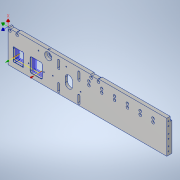
# Autodesk Inventor part: Frame Back
Saved by Autodesk Inventor 2020 (Build 240168000, 168)
## iProperties
Created: 2019-01-21
Part Number: Frame Back
Material: Aluminum 6061
Document SubType Name: Modeling
Designer: LillaHunden
Density: 2.7 g/cm^3
Appearance: Aluminum - Flat
Author: LillaHunden
Autodesk Inventor part; units mm, degrees
ref_plane "YZ Plane" through (0, 0, 0) normal (1, 0, 0) x (0, 1, 0)
ref_plane "XZ Plane" through (0, 0, 0) normal (0, 1, 0) x (-1, 0, 0)
sketch "Sketch1" plane through (0, 0, 0) normal (0, 0, 1) x (1, 0, 0)
  line L0 (-165.2266, -26.9823) -> (205.7734, -26.9823)
  line L1 (205.7734, -26.9823) -> (205.7734, -103.9647)
  line L2 (205.7734, -103.9647) -> (-165.2266, -103.9647)
  line L3 (-165.2266, -103.9647) -> (-165.2266, -26.9823)
  line L4 (15.7734, -103.9647) -> (41.2734, -103.9647) construction
  point P0 (0, 0)
  point P1 (20.2734, -103.9647)
  constraints: 8 end point, 2 parallel, 1 horizontal, 1 horizontal alignment, 1 midpoint, 1 perpendicular
extrude "Extrusion1" add sketch "Sketch1" along normal blind 12
sketch "Sketch2" plane through (-165.2266, -103.9647, 0) normal (-1, 0, 0) x (0, 0, 1)
  line L0 (0, 0) -> (0, 76.9823) construction
  line L1 (0, 0) -> (12, 0) projected
  line L2 (12, 76.9823) -> (12, 0) construction
  line L3 (0, 76.9823) -> (12, 76.9823) construction
  line L4 (4, 67) -> (-280, 67) construction
  line L5 (4, 67) -> (4, 76.9823) construction
  line L6 (-280, 76.9823) -> (4, 76.9823) construction
  line L7 (0, 103.9647) -> (4, 103.9647)
  line L8 (4, 103.9647) -> (4, 67)
  line L9 (4, 67) -> (0, 67)
  line L10 (0, 67) -> (0, 103.9647)
  line L11 (-280, 76.9823) -> (-280, 67) projected
  constraints: 8 end point, 2 parallel, 1 horizontal, 1 perpendicular, 1 other
extrude "Extrusion2" cut sketch "Sketch2" against normal through all
sketch "Sketch3" plane through (0, 0, 0) normal (0, 0, -1) x (-1, 0, 0)
  circle A0 centre (71.5266, -39.9823) radius 2.5 construction
  arc A1 (66.419, -43.1308) -> (56.0091, -36.9647) centre (56.0091, -48.8349) ccw
  line L0 (165.2266, -36.9647) -> (-205.7734, -36.9647) construction
  line L1 (71.5266, -34.9823) -> (71.5266, -45.9823) construction
  arc A2 (87.044, -36.9647) -> (76.6341, -43.1308) centre (87.044, -48.8349) ccw
  line L2 (56.0091, -36.9647) -> (87.044, -36.9647)
  arc A3 (66.419, -43.1308) -> (76.6341, -43.1308) centre (71.5266, -39.9823) ccw
  arc A4 (75.5133, -36.9647) -> (67.5399, -36.9647) centre (71.5266, -39.9823) ccw construction
  point P0 (0, 0)
  dimension "d9" = 6
  constraints: 10 point on circle, 5 centre point, 4 end point, 3 point on line, 3 symmetric about line, 2 tangent, 1 coincident, 1 collinear, 1 other
  measures "d9" radius of A3
extrude "Extrusion3" cut sketch "Sketch3" against normal up to surface (4 mm away)
sketch "Sketch4" plane through (0, 0, 0) normal (0, 0, -1) x (-1, 0, 0)
  circle A0 centre (23.2266, -67.9647) radius 18.9 projected
  circle A1 centre (23.2266, -67.9647) radius 19.5 projected
  point P0 (0, 0)
extrude "Extrusion4" cut sketch "Sketch4" against normal blind 6.25 contours A0 | A1
sketch "Sketch5" plane through (-23.2266, -67.9647, 6.25) normal (0, 0, -1) x (-1, 0, 0)
  circle A0 centre (0, 0) radius 2.5 projected
  circle A1 centre (0, 0) radius 3.5
  point P0 (-23.2266, 67.9647)
  dimension "d15" = 1
  constraints: 1 centre point
  measures "d15" radial gap between concentric circles of A0 A1
extrude "Extrusion5" cut sketch "Sketch5" against normal through all contours A0 | A1
sketch "Sketch6" plane through (0, 0, 0) normal (0, 0, -1) x (-1, 0, 0)
  circle A0 centre (-0.3434, -44.3947) radius 2.6 projected
  circle A1 centre (46.7966, -44.3947) radius 2.6 projected
  circle A2 centre (46.7966, -91.5347) radius 2.6 projected
  circle A3 centre (-0.3434, -91.5347) radius 2.6 projected
  point P0 (0, 0)
hole "Hole1" at (0.3434, -91.5347, 0) at (-46.7966, -91.5347, 0) at (0.3434, -44.3947, 0) at (-46.7966, -44.3947, 0) direction (0, 0, 1) diameter 4.134 depth 14.2 thread size "M5x0.8" class "6H" standard "ISO Metric profile"
chamfer "Chamfer3" distance 0.2 angle 45 8 edges at (0.3434, -46.4617, 12) (-46.7966, -46.4617, 12) (-46.7966, -93.6017, 12) (0.3434, -93.6017, 12) (0.3434, -93.6017, 0) (-46.7966, -93.6017, 0) (-46.7966, -46.4617, 0) (0.3434, -46.4617, 0)
sketch "Sketch7" plane through (-165.2266, -36.9647, 4) normal (0, 0, -1) x (-1, 0, 0)
  circle A0 centre (-93.7, -3.0177) radius 4.7625 projected
  circle A1 centre (-93.7, -3.0177) radius 4.7125
  point P0 (-165.2266, 36.9647)
  dimension "d31" = 0.05
  constraints: 1 centre point
  measures "d31" radial gap between concentric circles of A0 A1
extrude "Extrusion6" cut sketch "Sketch7" against normal through all contours A0 | A1
chamfer "Chamfer4" distance 0.5 angle 45 2 edges at (-66.7641, -39.9823, 4) (-66.7641, -39.9823, 12)
sketch "Sketch8" plane through (-165.2266, -36.9647, 4) normal (0, 0, -1) x (-1, 0, 0)
  line L0 (-18, 6.4823) -> (-7, 6.4823) construction
  line L1 (-7, 6.4823) -> (-7, 10.6239) construction
  line L2 (-18, 10.6239) -> (-18, 6.4823) construction
  line L3 (-19, 7.9823) -> (-6, 7.9823) projected
  line L4 (-19, 9.9823) -> (-19, 7.9823) projected
  line L5 (-6, 7.9823) -> (-6, 9.9823) projected
  arc A0 (-21.8284, 9.9823) -> (-19, 7.9823) centre (-19, 10.9823) ccw
  line L6 (-371, 9.9823) -> (0, 9.9823) projected
  line L7 (-21.8284, 9.9823) -> (-6, 9.9823)
  line L8 (-12.5, 7.9823) -> (-12.5, 13.9823)
  arc A1 (-6, 7.9823) -> (-3.1716, 9.9823) centre (-6, 10.9823) ccw
  line L9 (-3.1716, 9.9823) -> (-6, 9.9823)
  point P0 (-165.2266, 36.9647)
  dimension "d37" = 6
  constraints: 6 end point, 5 point on circle, 4 point on line, 2 centre point, 1 collinear, 1 midpoint, 1 perpendicular, 1 symmetric about line, 1 tangent, 1 vertical, 1 other
  measures "d37" diameter of A0
extrude "Extrusion7" cut sketch "Sketch8" against normal through all
sketch "Sketch9" plane through (-165.2266, -36.9647, 4) normal (0, 0, -1) x (-1, 0, 0)
  line L0 (-209, 9.9823) -> (-209, 7.9823) projected
  line L1 (-209, 7.9823) -> (-196, 7.9823) projected
  line L2 (-196, 7.9823) -> (-196, 9.9823) projected
  line L3 (-190, 9.9823) -> (-196, 9.9823) projected
  line L4 (-190, 0) -> (-190, 9.9823) projected
  line L5 (-215, 0) -> (-190, 0) projected
  line L6 (-215, 0) -> (-215, 9.9823) projected
  line L7 (-209, 9.9823) -> (-215, 9.9823) projected
  arc A0 (-211.8284, 9.9823) -> (-209, 7.9823) centre (-209, 10.9823) ccw
  line L8 (-202.5, 7.9823) -> (-202.5, 9.9823) construction
  arc A1 (-196, 7.9823) -> (-193.1716, 9.9823) centre (-196, 10.9823) ccw
  line L9 (-371, 9.9823) -> (-21.8284, 9.9823) projected
  line L10 (-211.8284, 9.9823) -> (-193.1716, 9.9823)
  point P0 (-165.2266, 36.9647)
  dimension "d40" = 6
  constraints: 5 end point, 5 point on circle, 3 point on line, 2 centre point, 2 midpoint, 1 symmetric about line, 1 tangent, 1 vertical, 1 other
  measures "d40" diameter of A0
extrude "Extrusion8" cut sketch "Sketch9" against normal through all contours L9 L2 L1 L0 | L0 A0 L7 | L3 A1 L2
sketch "Sketch10" plane through (0, 0, 0) normal (0, 0, -1) x (-1, 0, 0)
  circle A0 centre (23.2266, -67.9647) radius 3.5 construction
  line L0 (23.2266, -75.9647) -> (23.2266, -59.9647) construction
  line L1 (3.7266, -75.9647) -> (3.7266, -59.9647)
  line L2 (42.7266, -59.9647) -> (42.7266, -75.9647)
  arc A1 (3.7266, -75.9647) -> (42.7266, -75.9647) centre (23.2266, -75.9647) ccw
  arc A2 (42.7266, -59.9647) -> (3.7266, -59.9647) centre (23.2266, -59.9647) ccw
  circle A3 centre (23.2266, -67.9647) radius 3.5 construction
  circle A4 centre (23.2266, -67.9647) radius 19.5 construction
  line L3 (56.0091, -36.9647) -> (-205.7734, -36.9647) construction
  point P0 (0, 0)
  dimension "d43" = 8
  constraints: 8 end point, 5 tangent, 4 point on circle, 2 centre point, 1 midpoint, 1 parallel, 1 vertical
  measures "d43" distance of L0.end A0.centre
extrude "Extrusion9" cut sketch "Sketch10" against normal up to surface (6.25 mm away)
sketch "Sketch11" plane through (0, 0, 0) normal (0, 0, -1) x (-1, 0, 0)
  line L0 (-0.3434, -36.3947) -> (-0.3434, -52.3947) construction
  line L1 (-2.9434, -36.3947) -> (-2.9434, -52.3947)
  line L2 (2.2566, -52.3947) -> (2.2566, -36.3947)
  arc A0 (2.2566, -36.3947) -> (-2.9434, -36.3947) centre (-0.3434, -36.3947) ccw
  arc A1 (-2.9434, -52.3947) -> (2.2566, -52.3947) centre (-0.3434, -52.3947) ccw
  circle A2 centre (-0.3434, -44.3947) radius 2.067 construction
  circle A3 centre (46.7966, -44.3947) radius 2.267 construction
  line L3 (56.0091, -36.9647) -> (-205.7734, -36.9647) construction
  line L4 (46.7966, -36.3947) -> (46.7966, -52.3947) construction
  line L5 (44.1966, -36.3947) -> (44.1966, -52.3947)
  line L6 (49.3966, -52.3947) -> (49.3966, -36.3947)
  arc A4 (49.3966, -36.3947) -> (44.1966, -36.3947) centre (46.7966, -36.3947) ccw
  arc A5 (44.1966, -52.3947) -> (49.3966, -52.3947) centre (46.7966, -52.3947) ccw
  line L7 (-0.3434, -83.5347) -> (-0.3434, -99.5347) construction
  line L8 (-2.9434, -83.5347) -> (-2.9434, -99.5347)
  line L9 (2.2566, -99.5347) -> (2.2566, -83.5347)
  arc A6 (2.2566, -83.5347) -> (-2.9434, -83.5347) centre (-0.3434, -83.5347) ccw
  arc A7 (-2.9434, -99.5347) -> (2.2566, -99.5347) centre (-0.3434, -99.5347) ccw
  line L10 (46.7966, -83.5347) -> (46.7966, -99.5347) construction
  line L11 (44.1966, -83.5347) -> (44.1966, -99.5347)
  line L12 (49.3966, -99.5347) -> (49.3966, -83.5347)
  arc A8 (49.3966, -83.5347) -> (44.1966, -83.5347) centre (46.7966, -83.5347) ccw
  arc A9 (44.1966, -99.5347) -> (49.3966, -99.5347) centre (46.7966, -99.5347) ccw
  point P0 (0, 0)
  point P1 (46.7966, -44.3947)
  point P2 (46.7966, -44.3947)
  point P3 (-0.3434, -91.5347)
  point P4 (-0.3434, -91.5347)
  point P5 (46.7966, -91.5347)
  point P6 (46.7966, -91.5347)
  dimension "d46" = 8
  dimension "d47" = 5.2
  dimension "d50" = 47.14
  dimension "d53" = 47.14
  constraints: 32 end point, 16 point on circle, 8 centre point, 4 coincident, 4 tangent, 2 vertical, 1 collinear, 1 horizontal, 1 midpoint, 1 parallel, 38 other
  measures "d46" distance of point (-0.343, -44.395) L0.end
  measures "d47" diameter of A1
  measures "d50" distance of L1.start L5.start
  measures "d53" distance of L1.start L8.start
extrude "Extrusion10" cut sketch "Sketch11" against normal through all
sketch "Sketch12" plane through (0, 0, 6.25) normal (0, 0, -1) x (-1, 0, 0)
  circle A0 centre (23.2266, -67.9647) radius 3.5 construction
  line L0 (23.2266, -75.9647) -> (23.2266, -59.9647) construction
  circle A1 centre (23.2266, -67.9647) radius 3.5 construction
  line L1 (19.7266, -75.9647) -> (19.7266, -59.9647)
  line L2 (26.7266, -59.9647) -> (26.7266, -75.9647)
  arc A2 (19.7266, -75.9647) -> (26.7266, -75.9647) centre (23.2266, -75.9647) ccw
  arc A3 (26.7266, -59.9647) -> (19.7266, -59.9647) centre (23.2266, -59.9647) ccw
  point P0 (0, 0)
  dimension "d58" = 8
  constraints: 8 end point, 4 point on circle, 4 tangent, 2 centre point, 1 midpoint, 1 parallel, 1 vertical
  measures "d58" distance of A1.centre L0.end
extrude "Extrusion11" cut sketch "Sketch12" against normal through all
sketch "Sketch13" plane through (0, 0, 12) normal (0, 0, 1) x (1, 0, 0)
  line L0 (-146.2266, -26.9823) -> (-146.2266, -28.9823) construction
  line L1 (-146.2266, -28.9823) -> (-159.2266, -28.9823) construction
  line L2 (-159.2266, -28.9823) -> (-159.2266, -26.9823) construction
  line L3 (-165.2266, -26.9823) -> (-159.2266, -26.9823) construction
  line L4 (-165.2266, -36.9647) -> (-165.2266, -26.9823) construction
  line L5 (-140.2266, -36.9647) -> (-165.2266, -36.9647) construction
  line L6 (-140.2266, -36.9647) -> (-140.2266, -26.9823) construction
  line L7 (-146.2266, -26.9823) -> (-140.2266, -26.9823) construction
  line L8 (43.7734, -26.9823) -> (43.7734, -28.9823) construction
  line L9 (43.7734, -28.9823) -> (30.7734, -28.9823) construction
  line L10 (30.7734, -28.9823) -> (30.7734, -26.9823) construction
  line L11 (24.7734, -26.9823) -> (30.7734, -26.9823) construction
  line L12 (24.7734, -36.9647) -> (24.7734, -26.9823) construction
  line L13 (49.7734, -36.9647) -> (24.7734, -36.9647) construction
  line L14 (49.7734, -36.9647) -> (49.7734, -26.9823) construction
  line L15 (43.7734, -26.9823) -> (49.7734, -26.9823) construction
  circle A0 centre (-161.2266, -33.2125) radius 1.621 projected
  circle A1 centre (-144.2266, -33.2125) radius 1.621 projected
  point P0 (0, 0)
  point P1 (-161.2266, -33.2125)
  point P2 (-144.2266, -33.2125)
  point P3 (28.7734, -33.2125)
  point P4 (45.7734, -33.2125)
  dimension "d61" = 4
  dimension "d62" = 4
  dimension "d63" = 4
  dimension "d64" = 4
  constraints: 3 horizontal alignment
  measures "d61" distance from line of L4 point (-161.227, -33.213)
  measures "d62" distance from line of L6 point (-144.227, -33.213)
  measures "d63" distance from line of L12 point (28.773, -33.213)
  measures "d64" distance from line of L14 point (45.773, -33.213)
hole "Hole2" at (-161.2266, -33.2125, 12) at (-144.2266, -33.2125, 12) at (28.7734, -33.2125, 12) at (45.7734, -33.2125, 12) direction (0, 0, -1) diameter 3.4 depth 14.2 counterbore diameter 6.5 counterbore depth 3.4 clearance for "Socket Head Cap Screw ISO 4762" size "M3" standard "ISO"
sketch "Sketch14" plane through (0, 0, 12) normal (0, 0, 1) x (1, 0, 0)
  circle A0 centre (77.1068, -51.298) radius 1.621 construction
  circle A1 centre (173.6068, -51.298) radius 1.621 construction
  line L0 (108.2734, -36.9647) -> (108.2734, -41.9647) construction
  line L1 (108.2734, -41.9647) -> (93.2734, -41.9647) construction
  line L2 (93.2734, -41.9647) -> (93.2734, -36.9647) construction
  line L3 (12.7734, -36.9647) -> (93.2734, -36.9647) construction
  line L4 (12.7734, -55.9647) -> (12.7734, -36.9647) construction
  line L5 (205.7734, -55.9647) -> (12.7734, -55.9647) construction
  line L6 (205.7734, -55.9647) -> (205.7734, -36.9647) construction
  line L7 (108.2734, -36.9647) -> (205.7734, -36.9647) construction
  circle A2 centre (23.6068, -43.298) radius 1.621 projected
  circle A3 centre (53.6068, -51.298) radius 1.621 projected
  circle A4 centre (83.6068, -51.298) radius 1.621 projected
  circle A5 centre (113.6068, -43.298) radius 1.621 projected
  circle A6 centre (143.6068, -51.298) radius 1.621 projected
  circle A7 centre (173.6068, -43.298) radius 1.621 projected
  circle A8 centre (143.6068, -43.298) radius 1.621 projected
  circle A9 centre (113.6068, -51.298) radius 1.621 projected
  circle A10 centre (83.6068, -43.298) radius 1.621 projected
  circle A11 centre (53.6068, -43.298) radius 1.621 projected
  circle A12 centre (23.6068, -51.298) radius 1.621 projected
  point P0 (0, 0)
  point P1 (173.6068, -43.298)
  point P2 (143.6068, -51.298)
  point P3 (113.6068, -51.298)
  point P4 (83.6068, -51.298)
  point P5 (53.6068, -51.298)
  point P6 (23.6068, -51.298)
  point P7 (173.6068, -43.298)
  point P8 (143.6068, -43.298)
  point P9 (113.6068, -43.298)
  point P10 (83.6068, -43.298)
  point P11 (53.6068, -43.298)
  point P12 (23.6068, -43.298)
  dimension "d81" = 30
  dimension "d84" = 8
  constraints: 1 horizontal, 1 vertical, 11 other
  measures "d81" distance of A1.centre point (143.607, -51.298)
  measures "d84" distance of A1.centre point (173.607, -43.298)
hole "Hole3" at (173.6068, -43.298, 12) at (173.6068, -51.298, 12) at (143.6068, -51.298, 12) at (143.6068, -43.298, 12) at (113.6068, -51.298, 12) at (113.6068, -43.298, 12) at (83.6068, -43.298, 12) at (83.6068, -51.298, 12) at (53.6068, -51.298, 12) at (53.6068, -43.298, 12) at (23.6068, -51.298, 12) at (23.6068, -43.298, 12) direction (0, 0, -1) diameter 3.242 end through all counterbore diameter 6.5 counterbore depth 3.4 thread size "M4x0.7" class "6H" standard "ISO Metric profile"
sketch "Sketch15" plane through (0, 0, 0) normal (0, 0, -1) x (-1, 0, 0)
  line L0 (51.2266, -42.9647) -> (51.2266, -92.9647) construction
  line L1 (-4.7734, -92.9647) -> (-4.7734, -42.9647) construction
  line L2 (-1.7734, -39.9647) -> (48.2266, -39.9647) construction
  line L3 (-1.7734, -38.9647) -> (48.2266, -38.9647) construction
  line L4 (-5.7734, -92.9647) -> (-5.7734, -42.9647) construction
  line L5 (-10.1867, -31.4447) -> (56.6399, -31.4447)
  line L6 (56.6399, -31.4447) -> (56.6399, -107.0786)
  line L7 (56.6399, -107.0786) -> (-10.1867, -107.0786)
  line L8 (-10.1867, -107.0786) -> (-10.1867, -31.4447)
  line L9 (23.2266, -38.9647) -> (23.2266, -140.4412) construction
  line L10 (-205.7734, -103.9647) -> (165.2266, -103.9647) construction
  point P0 (0, 0)
  dimension "d87" = 1
  dimension "d88" = 1
  constraints: 14 end point, 4 parallel, 2 perpendicular, 1 horizontal, 1 midpoint, 1 other
  measures "d87" distance between parallel lines of L2 L3
  measures "d88" distance between parallel lines of L1 L4
extrude "Extrusion12" cut sketch "Sketch15" against normal blind 4
sketch "Sketch16" plane through (0, 0, 12) normal (0, 0, 1) x (1, 0, 0)
  arc A0 (-19.7266, -59.9647) -> (-26.7266, -59.9647) centre (-23.2266, -59.9647) ccw construction
  arc A1 (-26.7266, -75.9647) -> (-19.7266, -75.9647) centre (-23.2266, -75.9647) ccw construction
  circle A2 centre (-23.2266, -67.9647) radius 8 construction
  circle A3 centre (-23.2266, -67.9647) radius 8.6 construction
  line L0 (-23.2266, -53.9647) -> (-23.2266, -81.9647) construction
  line L1 (-31.8266, -62.5647) -> (-31.8266, -73.3647)
  line L2 (-14.6266, -73.3647) -> (-14.6266, -62.5647)
  arc A4 (-14.6266, -62.5647) -> (-31.8266, -62.5647) centre (-23.2266, -62.5647) ccw
  arc A5 (-31.8266, -73.3647) -> (-14.6266, -73.3647) centre (-23.2266, -73.3647) ccw
  arc A6 (-19.7266, -59.9647) -> (-26.7266, -59.9647) centre (-23.2266, -59.9647) ccw projected
  point P0 (0, 0)
  point P1 (-23.2266, -67.9647)
  point P2 (-23.2266, -79.4647)
  point P3 (-23.2266, -56.4647)
  dimension "d91" = 0.6
  dimension "d92" = 2.5
  dimension "d93" = 2.5
  constraints: 8 end point, 8 point on circle, 4 point on line, 4 tangent, 3 centre point, 1 midpoint, 1 parallel, 1 vertical
  measures "d91" radial gap between concentric circles of A2 A3
  measures "d92" distance of point (-23.227, -79.465) L0.end
  measures "d93" distance of point (-23.227, -56.465) L0.start
extrude "Extrusion13" cut sketch "Sketch16" against normal through all
sketch "Sketch17" plane through (0, 0, 12) normal (0, 0, 1) x (1, 0, 0)
  circle A0 centre (-71.5266, -39.9823) radius 8 construction
  circle A1 centre (-71.5266, -39.9823) radius 8.6
  point P0 (0, 0)
  dimension "d96" = 0.6
  constraints: 1 centre point
  measures "d96" radial gap between concentric circles of A0 A1
ref_plane "Work Plane1" through (-31.4029, -76.141, 6) normal (0, 0, -1) x (0.1439331, 0.9895874, 0)
extrude "Extrusion14" cut sketch "Sketch17" against normal up to surface (6 mm away)
sketch "Sketch18" plane through (-143.3981, -26.9823, 12) normal (0, 1, 0) x (1, 0, 0)
  line L0 (79.8716, -13.2) -> (63.8716, -13.2) construction
  line L1 (71.8716, -13.2) -> (71.8716, 7.5) construction
  line L2 (67.1091, 7.5) -> (76.6341, 7.5) construction
  line L3 (70.8561, 2.5) -> (71.8716, 2.5) construction
  circle A0 centre (71.8716, 2.5) radius 2
  line L4 (68.3716, 4) -> (68.3716, 1) projected
  point P0 (143.3981, 12)
  dimension "d99" = 4
  constraints: 4 end point, 2 midpoint, 1 centre point, 1 coincident, 1 perpendicular, 1 point on line
  measures "d99" diameter of A0
extrude "Extrusion15" cut sketch "Sketch18" against normal up to next
sketch "Sketch19" plane through (205.7734, -103.9647, 12) normal (1, 0, 0) x (0, 0, -1)
  point P0 (4.05, 68.9823)
  point P1 (4.05, 58.9823)
  point P2 (4.05, 43.4912)
  point P3 (4.05, 33.4912)
  point P4 (4.05, 18)
  point P5 (4.05, 8)
hole "Hole4" at (205.7734, -34.9823, 7.95) at (205.7734, -44.9823, 7.95) at (205.7734, -60.4735, 7.95) at (205.7734, -70.4735, 7.95) at (205.7734, -85.9647, 7.95) at (205.7734, -95.9647, 7.95) direction (-1, 0, 0) diameter 2.459 depth 8 tip angle 120 thread size "M3x0.5" class "6H" standard "ISO Metric profile"
sketch "Sketch20" plane through (-165.2266, -103.9647, 12) normal (-1, 0, 0) x (0, 0, 1)
  point P0 (-4.05, 58.9823)
  point P1 (-4.05, 43.4912)
  point P2 (-4.05, 33.4912)
  point P3 (-4.05, 18)
  point P4 (-4.05, 8)
hole "Hole6" at (-165.2266, -44.9823, 7.95) at (-165.2266, -60.4735, 7.95) at (-165.2266, -70.4735, 7.95) at (-165.2266, -85.9647, 7.95) at (-165.2266, -95.9647, 7.95) direction (1, 0, 0) diameter 2.459 depth 8 tip angle 120 thread size "M3x0.5" class "6H" standard "ISO Metric profile"
sketch "Sketch21" plane through (0, 0, 12) normal (0, 0, 1) x (1, 0, 0)
  line L0 (-110.2766, -61.1147) -> (-88.5766, -61.1147) construction
  line L1 (-85.5766, -64.1147) -> (-85.5766, -90.4147) construction
  arc A0 (-85.5766, -64.1147) -> (-88.5766, -61.1147) centre (-88.5766, -64.1147) ccw construction
  arc A1 (-110.2766, -61.1147) -> (-113.2766, -64.1147) centre (-110.2766, -64.1147) ccw construction
  line L2 (-145.2766, -90.4147) -> (-145.2766, -64.1147) construction
  line L3 (-88.5766, -93.4147) -> (-110.2766, -93.4147) construction
  arc A2 (-88.5766, -93.4147) -> (-85.5766, -90.4147) centre (-88.5766, -90.4147) ccw construction
  line L4 (-117.5766, -64.1147) -> (-117.5766, -90.4147) construction
  arc A3 (-113.2766, -90.4147) -> (-110.2766, -93.4147) centre (-110.2766, -90.4147) ccw construction
  arc A4 (-85.5766, -64.1147) -> (-88.5766, -61.1147) centre (-88.5766, -64.1147) ccw construction
  line L5 (-110.2766, -61.1147) -> (-88.5766, -61.1147) construction
  arc A5 (-110.2766, -61.1147) -> (-113.2766, -64.1147) centre (-110.2766, -64.1147) ccw construction
  arc A6 (-85.5766, -64.1147) -> (-88.5766, -61.1147) centre (-88.5766, -64.1147) ccw construction
  line L6 (-110.2766, -61.1147) -> (-88.5766, -61.1147) construction
  arc A7 (-85.5766, -64.1147) -> (-88.5766, -61.1147) centre (-88.5766, -64.1147) ccw construction
  arc A8 (-110.2766, -61.1147) -> (-113.2766, -64.1147) centre (-110.2766, -64.1147) ccw construction
  line L7 (-110.2766, -61.1147) -> (-88.5766, -61.1147)
  line L8 (-85.5766, -90.4147) -> (-85.5766, -64.1147)
  line L9 (-113.2766, -90.4147) -> (-113.2766, -64.1147) construction
  arc A9 (-110.7168, -61.9591) -> (-112.4321, -63.6745) centre (-110.2766, -64.1147) ccw construction
  line L10 (-113.2766, -64.1147) -> (-113.2766, -91.2147)
  arc A10 (-113.2766, -91.2147) -> (-110.7766, -93.7147) centre (-110.7766, -91.2147) ccw
  line L11 (-110.7766, -93.7147) -> (-88.0766, -93.7147)
  arc A11 (-88.0766, -93.7147) -> (-85.5766, -91.2147) centre (-88.0766, -91.2147) ccw
  line L12 (-85.5766, -91.2147) -> (-85.5766, -64.1147)
  arc A12 (-85.5766, -64.1147) -> (-88.5766, -61.1147) centre (-88.5766, -64.1147) ccw
  arc A13 (-110.2766, -61.1147) -> (-113.2766, -64.1147) centre (-110.2766, -64.1147) ccw
  point P0 (0, 0)
  dimension "d119" = 2.2
  constraints: 12 end point, 11 point on circle, 7 tangent, 5 centre point, 3 equal length, 2 concentric, 1 perpendicular, 1 point on line
  measures "d119" radius of A9
extrude "Extrusion16" cut sketch "Sketch21" against normal through all
chamfer "Chamfer5" distance 0.5 angle 45 7 edges at (-86.4552, -61.9933, 12) (-85.5766, -77.6647, 12) (-86.3088, -92.9824, 12) (-99.4266, -93.7147, 12) (-112.5443, -92.9824, 12) (-113.2766, -77.6647, 12) (-112.3979, -61.9933, 12)
sketch "Sketch22" plane through (0, 0, 12) normal (0, 0, 1) x (1, 0, 0)
  circle A0 centre (-117.4266, -77.2647) radius 2.1 construction
  circle A1 centre (-81.4266, -77.2647) radius 2.1 construction
  point P0 (0, 0)
hole "Hole9" at (-117.4266, -77.2647, 12) at (-81.4266, -77.2647, 12) direction (0, 0, -1) diameter 2.459 end through all thread size "M3x0.5" class "6H" standard "ISO Metric profile"
sketch "Sketch24" plane through (0, 0, 12) normal (0, 0, 1) x (1, 0, 0)
  line L0 (-130.5156, -91.1647) -> (-140.7656, -91.1647) construction
  line L1 (-141.6656, -91.1647) -> (-151.9156, -91.1647) construction
  line L2 (-152.1156, -90.9647) -> (-152.1156, -62.3647) construction
  line L3 (-151.9156, -62.1647) -> (-141.8656, -62.1647) construction
  line L4 (-140.7656, -62.1647) -> (-130.5156, -62.1647) construction
  line L5 (-130.3156, -62.3647) -> (-130.3156, -90.9647) construction
  line L6 (-152.1156, -62.3647) -> (-130.5156, -62.3647) construction
  line L7 (-130.5156, -62.3647) -> (-130.5156, -90.9647) construction
  line L8 (-130.5156, -90.9647) -> (-152.1156, -90.9647) construction
  line L9 (-152.1156, -90.9647) -> (-152.1156, -62.3647) construction
  line L10 (-130.0156, -91.4647) -> (-130.0156, -61.8647)
  line L11 (-130.0156, -61.8647) -> (-152.6156, -61.8647)
  line L12 (-152.6156, -61.8647) -> (-152.6156, -91.4647)
  line L13 (-152.6156, -91.4647) -> (-130.0156, -91.4647)
  point P0 (0, 0)
  dimension "d140" = 0.5
  constraints: 16 end point, 4 parallel, 2 perpendicular, 1 horizontal, 1 point on line, 3 other
  measures "d140" distance between parallel lines of L7 L10
extrude "Extrusion17" cut sketch "Sketch24" against normal through all
sketch "Sketch25" plane through (0, 0, 12) normal (0, 0, 1) x (1, 0, 0)
  circle A0 centre (-151.166, -90.0151) radius 2.05
  line L0 (-152.6156, -91.4647) -> (-152.6156, -61.8647) construction
  line L1 (-130.0156, -91.4647) -> (-152.6156, -91.4647) construction
  line L2 (-130.0156, -61.8647) -> (-130.0156, -91.4647) construction
  line L3 (-152.6156, -61.8647) -> (-130.0156, -61.8647) construction
  line L4 (-152.6156, -91.4647) -> (-145.9755, -84.8246) construction
  circle A1 centre (-131.4651, -90.0151) radius 2.05
  circle A2 centre (-131.4651, -63.3142) radius 2.05
  circle A3 centre (-151.166, -63.3142) radius 2.05
  line L5 (-152.6156, -61.8647) -> (-147.7303, -66.7499) construction
  line L6 (-130.0156, -61.8647) -> (-136.8881, -68.7372) construction
  line L7 (-130.0156, -91.4647) -> (-137.3176, -84.1626) construction
  point P0 (0, 0)
  dimension "d143" = 4.1
  dimension "d145" = 4.1
  dimension "d146" = 4.1
  dimension "d147" = 4.1
  dimension "d144" = 45
  dimension "d148" = 45
  dimension "d149" = 45
  dimension "d150" = 45
  constraints: 8 end point, 4 coincident, 4 point on line, 12 other
  measures "d144" angle of L1 L4
  measures "d148" angle of L2 L6
  measures "d149" angle of L0 L5
  measures "d150" angle of L1 L7
extrude "Extrusion18" cut sketch "Sketch25" against normal through all
fillet "Fillet1" radius 2 8 edges at (-130.0156, -88.5655, 6) (-132.9147, -91.4647, 6) (-149.7164, -91.4647, 6) (-152.6156, -88.5655, 6) (-152.6156, -64.7638, 6) (-149.7164, -61.8647, 6) (-132.9147, -61.8647, 6) (-130.0156, -64.7638, 6)
chamfer "Chamfer6" distance 0.5 angle 45 16 edges at (-141.3156, -61.8647, 12) (-133.0426, -61.7891, 12) (-130.0156, -61.8647, 12) (-129.94, -64.8917, 12) (-130.0156, -76.6647, 12) (-129.94, -88.4376, 12) (-130.0156, -91.4647, 12) (-133.0426, -91.5402, 12) (-141.3156, -91.4647, 12) (-149.5885, -91.5402, 12) (-152.6156, -91.4647, 12) (-152.6911, -88.4376, 12) (-152.6156, -76.6647, 12) (-152.6911, -64.8917, 12) (-152.6156, -61.8647, 12) (-149.5885, -61.7891, 12)
sketch "Sketch26" plane through (0, 0, 12) normal (0, 0, 1) x (1, 0, 0)
  circle A0 centre (-94.1611, -39.8647) radius 3.5 construction
  circle A1 centre (-29.1186, -39.8647) radius 3.5 construction
  circle A2 centre (4.2603, -74.0803) radius 3.5 construction
  circle A3 centre (-60.7822, -74.0803) radius 3.5 construction
  point P0 (0, 0)
hole "Hole10" at (-94.1611, -39.8647, 12) at (-29.1186, -39.8647, 12) at (-60.7822, -74.0803, 12) at (4.2603, -74.0803, 12) direction (0, 0, -1) diameter 2.459 end through all thread size "M3x0.5" class "6H" standard "ISO Metric profile"
body "Solid1"
